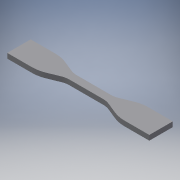
# Autodesk Inventor part: testSpecimen
Saved by Autodesk Inventor 2016 (Build 200138000, 138)
## iProperties
Created: 2017-01-10
Part Number: testSpecimen
Material: Generic
Document SubType Name: Modeling
Designer: Smoothie
Density: 1 g/cm^3
Appearance: Default
Author: Smoothie
Autodesk Inventor part; units mm, degrees
ref_plane "YZ Plane" through (0, 0, 0) normal (1, 0, 0) x (0, 1, 0)
ref_plane "XZ Plane" through (0, 0, 0) normal (0, 1, 0) x (-1, 0, 0)
ref_plane "XY Plane" through (0, 0, 0) normal (0, 0, 1) x (1, 0, 0)
sketch "Sketch1" plane through (0, 0, 0) normal (0, 0, 1) x (1, 0, 0)
  line L0 (57.5, -9.5) -> (-57.5, -9.5)
  line L1 (-57.5, -9.5) -> (-57.5, 9.5)
  line L2 (-57.5, 9.5) -> (57.5, 9.5)
  line L3 (57.5, 9.5) -> (57.5, -9.5)
  line L4 (57.5, -9.5) -> (-57.5, 9.5) construction
  line L5 (-57.5, -9.5) -> (57.5, 9.5) construction
  line L6 (12.5, -3) -> (-12.5, -3)
  line L7 (-12.5, -3) -> (-12.5, 3)
  line L8 (-12.5, 3) -> (12.5, 3)
  line L9 (12.5, 3) -> (12.5, -3)
  line L10 (12.5, -3) -> (-12.5, 3) construction
  line L11 (-12.5, -3) -> (12.5, 3) construction
  line L12 (16.5, -3) -> (-16.5, -3)
  line L13 (-16.5, -3) -> (-16.5, 3)
  line L14 (-16.5, 3) -> (16.5, 3)
  line L15 (16.5, 3) -> (16.5, -3)
  line L16 (16.5, -3) -> (-16.5, 3) construction
  line L17 (-16.5, -3) -> (16.5, 3) construction
  line L18 (32.5, -9.5) -> (-32.5, -9.5)
  line L19 (-32.5, -9.5) -> (-32.5, 9.5)
  line L20 (-32.5, 9.5) -> (32.5, 9.5)
  line L21 (32.5, 9.5) -> (32.5, -9.5)
  line L22 (32.5, -9.5) -> (-32.5, 9.5) construction
  line L23 (-32.5, -9.5) -> (32.5, 9.5) construction
  line L24 (-16.5, 9.5) -> (-16.5, -9.5)
  line L25 (16.5, -9.5) -> (16.5, 9.5)
  line L26 (-16.5, 3) -> (-32.5, 9.5)
  line L27 (-32.5, -9.5) -> (-16.5, -3)
  line L28 (16.5, 3) -> (32.5, 9.5)
  line L29 (16.5, -3) -> (32.5, -9.5)
  point P0 (0, 0)
  point P1 (0, 0)
  dimension "d0" = 115
  dimension "d1" = 19
  dimension "d2" = 6
  dimension "d3" = 25
  dimension "d4" = 33
  dimension "d5" = 65
  constraints: 60 end point, 10 midpoint, 8 parallel, 6 perpendicular, 5 point on line, 4 horizontal, 2 vertical alignment, 1 horizontal alignment
  measures "d0" distance of L0.start L0.end
  measures "d1" distance of L2.end L0.start
  measures "d2" distance of L6.end L7.end
  measures "d3" distance of L7.end L8.end
  measures "d4" distance of L12.start L12.end
  measures "d5" distance of L19.end L20.end
extrude "Extrusion1" add sketch "Sketch1" along normal blind 4 contours L0 L21 L2 L3 | L29 L15 L28 L21 | L12 L9 L14 L15 | L6 L7 L8 L9 | L0 L1 L2 L19 | L19 L26 L13 L27 | L13 L14 L7 L12
fillet "Fillet1" radius 25 4 edges at (-32.5, 9.5, 2) (-32.5, -9.5, 2) (32.5, 9.5, 2) (32.5, -9.5, 2)
fillet "Fillet2" radius 14 4 edges at (-16.5, 3, 2) (-16.5, -3, 2) (16.5, -3, 2) (16.5, 3, 2)
body "Solid1"
